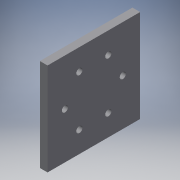
# Autodesk Inventor part: PlateForConnectionToArm
Saved by Autodesk Inventor 2016 SP1 (Build 200210100, 210)
## iProperties
Created: 2016-01-26
Part Number: PlateForConnectionToArm
Material: Generic
Document SubType Name: Modeling
Designer: steele
Density: 1 g/cm^3
Appearance: Default
Author: steele
Autodesk Inventor part; units mm, degrees
ref_plane "YZ Plane" through (0, 0, 0) normal (1, 0, 0) x (0, 1, 0)
ref_plane "XZ Plane" through (0, 0, 0) normal (0, 1, 0) x (-1, 0, 0)
ref_plane "XY Plane" through (0, 0, 0) normal (0, 0, 1) x (1, 0, 0)
sketch "Sketch1" plane through (0, 0, 0) normal (1, 0, 0) x (0, 1, 0)
  line L0 (-38.1, 38.1) -> (-38.1, -38.1)
  line L1 (-38.1, -38.1) -> (38.1, -38.1)
  line L2 (38.1, -38.1) -> (38.1, 38.1)
  line L3 (38.1, 38.1) -> (-38.1, 38.1)
  line L4 (-38.1, 38.1) -> (38.1, -38.1) construction
  line L5 (-38.1, -38.1) -> (38.1, 38.1) construction
  point P0 (0, 0)
  dimension "d0" = 76.2
  dimension "d1" = 76.2
  constraints: 12 end point, 2 midpoint, 2 parallel, 1 perpendicular, 1 vertical
  measures "d0" distance of L2.end L0.start
  measures "d1" distance of L1.end L2.end
extrude "Extrusion1" add sketch "Sketch1" against normal blind 6.35
sketch "Sketch4" plane through (-6.35, 0, 0) normal (-1, 0, 0) x (0, 0, 1)
  circle A0 centre (0, -23.8125) radius 2.54
  circle A1 centre (20.6222, -11.9063) radius 2.54
  circle A2 centre (20.6222, 11.9062) radius 2.54
  circle A3 centre (0, 23.8125) radius 2.54
  circle A4 centre (-20.6222, 11.9063) radius 2.54
  circle A5 centre (-20.6222, -11.9062) radius 2.54
  point P0 (0, 0)
  dimension "d13" = 5.08
  dimension "d14" = 23.8125
  dimension "d17" = 360
  constraints: 6 centre point, 13 other
  measures "d13" diameter of A0
  measures "d14" distance of A0.centre point (0, 0)
extrude "Extrusion3" cut sketch "Sketch4" against normal through all
sketch "Sketch5" plane through (-6.35, 0, 0) normal (-1, 0, 0) x (0, 0, 1)
  circle A0 centre (0, 0) radius 5
  dimension "d21" = 10
  constraints: 1 centre point, 1 coincident
  measures "d21" diameter of A0
extrude "Extrusion4" cut sketch "Sketch5" against normal through all
equation "\"d13\" = amHubBoltDiam"
equation "\"d14\" = 0.5 * amHubBoltHoleDiam"
equation "\"d21\" = centerHoleDiam"
equation "\"amHubBoltHoleDiam\" = 47.625"
equation "\"amHubBoltDiam\" = 5.08"
equation "\"centerHoleDiam\" = 10"
body "Solid1"
